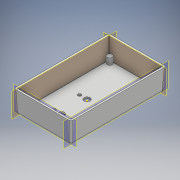
# Autodesk Inventor part: box_bottom
Saved by Autodesk Inventor 2018 (Build 220112000, 112)
## iProperties
Created: 2017-12-11
Part Number: box_bottom
Material: Generic
Document SubType Name: Modeling
Designer: caleb
Density: 1 g/cm^3
Appearance: Default
Author: caleb
Autodesk Inventor part; units mm, degrees
ref_plane "YZ Plane" through (0, 0, 0) normal (1, 0, 0) x (0, 1, 0)
ref_plane "XZ Plane" through (0, 0, 0) normal (0, 1, 0) x (-1, 0, 0)
ref_plane "XY Plane" through (0, 0, 0) normal (0, 0, 1) x (1, 0, 0)
sketch "Sketch1" plane through (0, 0, 0) normal (0, 0, 1) x (1, 0, 0)
  line L0 (-30, -50) -> (30, -50)
  line L1 (30, -50) -> (30, 50)
  line L2 (30, 50) -> (-30, 50)
  line L3 (-30, 50) -> (-30, -50)
  line L4 (-30, -50) -> (30, 50) construction
  line L5 (30, -50) -> (-30, 50) construction
  point P0 (0, 0)
  dimension "d0" = 100
  dimension "d1" = 60
  constraints: 12 end point, 2 midpoint, 2 parallel, 1 horizontal, 1 perpendicular
  measures "d0" distance of L0.end L1.end
  measures "d1" distance of L1.end L2.end
extrude "Extrusion1" add sketch "Sketch1" against normal blind 23 draft -3
fillet "Fillet1" radius 2 8 edges at (29.3973, 49.3973, -11.5) (28.7946, 0, -23) (0, 48.7946, -23) (-29.3973, 49.3973, -11.5) (-28.7946, 0, -23) (-29.3973, -49.3973, -11.5) (0, -48.7946, -23) (29.3973, -49.3973, -11.5)
shell "Shell1" thickness 1.75 removed faces 1 at (10, 16.0009, 0)
sketch "Sketch2" plane through (-26.8967, -46.8967, -21.25) normal (0, 0, 1) x (1, 0, 0)
  line L0 (0, 0) -> (53.7934, 0) construction
  line L1 (53.7934, 0) -> (53.7934, 93.7934) construction
  line L2 (53.7934, 93.7934) -> (0, 93.7934) construction
  line L3 (0, 93.7934) -> (0, 0) construction
  line L4 (3.0842, 2.4467) -> (50.7092, 2.4467) construction
  line L5 (50.7092, 2.4467) -> (50.7092, 91.3467) construction
  line L6 (54.043, 93.7934) -> (54.043, 0) construction
  circle A0 centre (3.0842, 91.3467) radius 2.675
  circle A1 centre (50.7092, 91.3467) radius 2.675
  circle A2 centre (50.7092, 2.4467) radius 2.675
  circle A3 centre (3.0842, 2.4467) radius 2.675
  point P0 (26.8967, 46.8967)
  point P1 (50.7092, 46.8967)
  point P2 (54.043, 46.8967)
  point P3 (26.8967, 2.4467)
  dimension "d6" = 47.625
  dimension "d7" = 88.9
  dimension "d8" = 5.35
  constraints: 4 centre point, 4 coincident, 4 end point, 3 equal radius, 3 horizontal alignment, 3 midpoint, 3 vertical alignment, 1 horizontal, 1 perpendicular
  measures "d6" distance of L4.end L4.start
  measures "d7" distance of L5.end L4.end
  measures "d8" diameter of A3
extrude "Extrusion2" add sketch "Sketch2" along normal blind 6.75
sketch "Sketch3" plane through (0, 0, -23) normal (0, 0, -1) x (-1, 0, 0)
  line L0 (26.8967, -46.8967) -> (-26.8967, -46.8967) construction
  line L1 (26.8967, 46.8967) -> (26.8967, -46.8967) construction
  line L2 (-26.8967, 46.8967) -> (26.8967, 46.8967) construction
  line L3 (-26.8967, -46.8967) -> (-26.8967, 46.8967) construction
  circle A0 centre (-11.6412, -41.6312) radius 2.885 construction
  circle A1 centre (2.7521, -27.0199) radius 3.429 construction
  circle A2 centre (-16.2979, -27.0199) radius 3.429 construction
  circle A3 centre (-16.2979, -0.3499) radius 3.429 construction
  circle A4 centre (2.7521, -0.3499) radius 3.429 construction
  line L4 (11.2743, 1.0471) -> (9.9911, 1.0471) construction
  line L5 (9.9911, 1.0471) -> (9.9911, -1.7469) construction
  line L6 (9.9911, -1.7469) -> (11.2743, -1.7469) construction
  arc A5 (11.2743, -1.7469) -> (11.2743, 1.0471) centre (2.7521, -0.3499) ccw construction
  line L7 (11.2743, -25.6229) -> (9.9911, -25.6229) construction
  line L8 (9.9911, -25.6229) -> (9.9911, -28.4169) construction
  line L9 (9.9911, -28.4169) -> (11.2743, -28.4169) construction
  arc A6 (11.2743, -28.4169) -> (11.2743, -25.6229) centre (2.7521, -27.0199) ccw construction
  line L10 (-7.7757, -25.6229) -> (-9.0589, -25.6229) construction
  line L11 (-9.0589, -25.6229) -> (-9.0589, -28.4169) construction
  line L12 (-9.0589, -28.4169) -> (-7.7757, -28.4169) construction
  arc A7 (-7.7757, -28.4169) -> (-7.7757, -25.6229) centre (-16.2979, -27.0199) ccw construction
  line L13 (-7.7757, 1.0471) -> (-9.0589, 1.0471) construction
  line L14 (-9.0589, 1.0471) -> (-9.0589, -1.7469) construction
  line L15 (-9.0589, -1.7469) -> (-7.7757, -1.7469) construction
  arc A8 (-7.7757, -1.7469) -> (-7.7757, 1.0471) centre (-16.2979, -0.3499) ccw construction
  point P0 (0, 0)
  point P1 (10.6327, -27.0199)
  point P2 (-8.4173, -27.0199)
  point P3 (-8.4173, -0.3499)
  point P4 (10.6327, -0.3499)
  point P5 (10.6327, -25.6229)
  point P6 (-8.4173, -25.6229)
  constraints: 5 coincident, 4 horizontal alignment, 4 vertical alignment, 2 midpoint
hole "Hole1" at (11.6412, -41.6312, -23) at (16.2979, -27.0199, -23) at (16.2979, -0.3499, -23) at (-2.7521, -0.3499, -23) at (-2.7521, -27.0199, -23) direction (0, 0, 1) diameter 6.35 end through all
hole "Hole2" at (-10.6327, -27.0199, -23) at (8.4173, -27.0199, -23) at (8.4173, -0.3499, -23) at (-10.6327, -0.3499, -23) direction (0, 0, 1) diameter 3.5 end through all
sketch "Sketch4" plane through (0, 0, -23) normal (0, 0, -1) x (-1, 0, 0)
  circle A0 centre (-11.6412, -41.6312) radius 3.175 projected
  point P0 (0, 0)
  point P1 (1.0588, -41.6312)
  dimension "d26" = 12.7
  constraints: 1 horizontal alignment
  measures "d26" distance of point (1.059, -41.631) A0.centre
hole "Hole3" at (-1.0588, -41.6312, -23) direction (0, 0, 1) diameter 5 end through all
ref_plane "Work Plane1" through (-27.1463, 25, -21.0131) normal (1, 0, 0) x (0, 1, 0)
ref_plane "Work Plane2" through (27.1463, -25, -21.0131) normal (-1, 0, 0) x (0, -1, 0)
ref_plane "Work Plane3" through (15, 47.1463, -21.0131) normal (0, -1, 0) x (1, 0, 0)
ref_plane "Work Plane4" through (-15, -47.1463, -21.0131) normal (0, 1, 0) x (-1, 0, 0)
body "Solid1"
